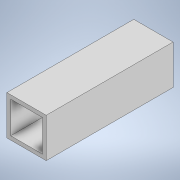
# Autodesk Inventor part: enclosure_80x25x25_mm
Saved by Autodesk Inventor 2020.2 (Build 242310000, 310)
## iProperties
Created: 2020-09-26
Part Number: enclosure_80x25x25_mm
Material: Generic
Document SubType Name: Modeling
Designer: Krishna Makhija
Density: 1 g/cm^3
Appearance: Default
Author: Krishna Makhija
Autodesk Inventor part; units mm, degrees
ref_plane "YZ Plane" through (0, 0, 0) normal (1, 0, 0) x (0, 1, 0)
ref_plane "XZ Plane" through (0, 0, 0) normal (0, 1, 0) x (-1, 0, 0)
ref_plane "XY Plane" through (0, 0, 0) normal (0, 0, 1) x (1, 0, 0)
sketch "Sketch1" plane through (0, 0, 0) normal (0, 0, 1) x (1, 0, 0)
  line L0 (-9.9998, 10.0001) -> (9.9998, 10.0001)
  line L1 (9.9998, 10.0001) -> (9.9998, -10.0001)
  line L2 (9.9998, -10.0001) -> (-9.9998, -10.0001)
  line L3 (-9.9998, -10.0001) -> (-9.9998, 10.0001)
  line L4 (-9.9998, 10.0001) -> (9.9998, -10.0001) construction
  line L5 (9.9998, 10.0001) -> (-9.9998, -10.0001) construction
  line L6 (-12.4001, 12.4005) -> (12.4001, 12.4005)
  line L7 (12.4001, 12.4005) -> (12.4001, -12.4005)
  line L8 (12.4001, -12.4005) -> (-12.4001, -12.4005)
  line L9 (-12.4001, -12.4005) -> (-12.4001, 12.4005)
  line L10 (-12.4001, 12.4005) -> (12.4001, -12.4005) construction
  line L11 (12.4001, 12.4005) -> (-12.4001, -12.4005) construction
  point P0 (0, 0)
  constraints: 24 end point, 4 midpoint, 4 parallel, 2 horizontal, 2 perpendicular
extrude "Extrusion1" add sketch "Sketch1" along normal blind 80
body "Solid1"
